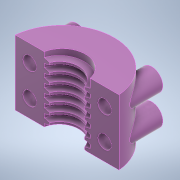
# Autodesk Inventor part: SpindleAdaptor_B_V3
Saved by Autodesk Inventor 2022.2 (Build 262287000, 287)
## iProperties
Created: 2022-11-20
Part Number: SpindleAdaptor_B_V3
Material: ABS Plastic
Document SubType Name: Modeling
Designer: jaege
Density: 1.06 g/cm^3
Appearance: Smooth - Purple
Mass: 4.16051 g
Surface Area: 27.1261 cm^2
Volume: 4.16051 cm^3
Author: jaege
Autodesk Inventor part; units mm, degrees
ref_plane "YZ Plane" through (0, 0, 0) normal (1, 0, 0) x (0, 1, 0)
ref_plane "XZ Plane" through (0, 0, 0) normal (0, 1, 0) x (-1, 0, 0)
ref_plane "XY Plane" through (0, 0, 0) normal (0, 0, 1) x (1, 0, 0)
sketch "Sketch1" plane through (0, 0, 0) normal (0, 1, 0) x (-1, 0, 0)
  circle A0 centre (0, 0) radius 12
  dimension "d0" = 24
  constraints: 1 centre point, 1 coincident
  measures "d0" diameter of A0
extrude "Extrusion1" add sketch "Sketch1" along normal blind 30
sketch "Sketch2" plane through (0, 30, 0) normal (0, 1, 0) x (1, 0, 0)
  circle A0 centre (0, 0) radius 5.25
  dimension "d3" = 10.5
  constraints: 1 centre point, 1 coincident
  measures "d3" diameter of A0
extrude "Extrusion2" cut sketch "Sketch2" against normal blind 15
sketch "Sketch3" plane through (0, 0, 0) normal (0, 0, 1) x (1, 0, 0)
  line L0 (12, 30) -> (-12, 30) projected
  line L1 (12, 0) -> (-12, 0) projected
  line L2 (-5.25, 15) -> (5.25, 15) projected
  line L3 (-5.25, 30) -> (5.25, 30) projected
  line L4 (-5.25, 30) -> (-5.25, 15) projected
  line L5 (5.25, 30) -> (5.25, 15) construction
  line L6 (-5.25, 15) -> (5.25, 15) projected
  line L7 (-4, 15) -> (4, 15) construction
  line L8 (4, 15) -> (4, 30) construction
  line L9 (4, 30) -> (-4, 30) construction
  line L10 (-4, 30) -> (-4, 15) construction
  line L11 (5.25, 30) -> (4, 29.6651)
  line L12 (2.634, 29.299) -> (4, 28.933) construction
  line L13 (4, 29.6651) -> (4, 28.933)
  line L14 (5.25, 28.5981) -> (5.25, 28)
  line L15 (5.25, 28) -> (4, 27.6651)
  line L16 (2.634, 27.299) -> (4, 26.933) construction
  line L17 (4, 29.6651) -> (2.634, 29.299) construction
  line L18 (4, 27.6651) -> (2.634, 27.299) construction
  line L19 (4, 28.933) -> (5.25, 28.5981)
  line L20 (4, 26.933) -> (5.25, 26.5981)
  line L21 (4, 27.6651) -> (4, 26.933)
  line L22 (5.25, 30) -> (5.25, 28.5981)
  line L23 (0, 30) -> (0, 15)
  point P0 (0, 0)
  point P1 (4, 29.299)
  dimension "d6" = 8
  dimension "d7" = 30
  dimension "d8" = 30
  dimension "d9" = 1.25
  dimension "d10" = 105
  dimension "d11" = 105
  dimension "d12" = 0.732
  dimension "d13" = 0.5981
  constraints: 34 end point, 9 point on line, 6 collinear, 3 midpoint, 2 parallel, 2 vertical, 1 horizontal, 1 perpendicular, 1 vertical alignment
  measures "d6" distance between parallel lines of L8 L10
  measures "d7" angle of L12 L11
  measures "d8" angle of L16 L15
  measures "d9" distance between parallel lines of L5 L13
  measures "d10" angle of L5 L11
  measures "d11" angle of L14 L15
  measures "d12" distance of L13.start L12.end
  measures "d13" distance of L14.start L14.end
coil "Coil1" sketch "Sketch3" operation add axis through (0, 30, 0) along (0, -1, 0) pitch 2 turns 7 hand right contours L22 L19 L13 L11
sketch "Sketch4" plane through (0, 0, 0) normal (0, -1, 0) x (1, 0, 0)
  circle A0 centre (0, 0) radius 2
  line L0 (-2, -2) -> (2, -2)
  line L1 (2, -2) -> (2, 1.5)
  line L2 (2, 1.5) -> (-2, 1.5)
  line L3 (-2, 1.5) -> (-2, -2)
  point P0 (1.3229, 1.5)
  point P1 (-1.3229, 1.5)
  dimension "d22" = 4
  dimension "d23" = 3.5
  constraints: 8 end point, 3 tangent, 2 parallel, 1 centre point, 1 coincident, 1 horizontal, 1 perpendicular
  measures "d22" diameter of A0
  measures "d23" distance of L0.end L1.end
extrude "Extrusion3" cut sketch "Sketch4" against normal blind 10 contours A0 L2 picked at (0.2249, -0.4939)
sketch "Sketch5" plane through (0, 0, 0) normal (0, 0, 1) x (1, 0, 0)
  line L0 (12, 30) -> (-12, 30) projected
  line L1 (-5.25, 15) -> (5.25, 15) projected
  line L2 (0, -6) -> (0, 36) projected
  line L3 (-8.625, 26) -> (-12, 26) construction
  line L4 (-8.625, 26) -> (-5.25, 26) construction
  line L5 (-5.25, 30) -> (-5.25, 15) projected
  line L6 (-12, 0) -> (-12, 30) projected
  circle A0 centre (-8.625, 19) radius 1.55
  circle A1 centre (-8.625, 26) radius 1.55
  circle A2 centre (8.625, 26) radius 1.55
  circle A3 centre (8.625, 19) radius 1.55
  point P0 (0, 0)
  point P1 (1.5921, 15)
  dimension "d26" = 4
  dimension "d27" = 4
  dimension "d28" = 3.1
  constraints: 4 centre point, 4 coincident, 4 end point, 4 vertical alignment, 3 equal radius, 2 horizontal, 2 horizontal alignment, 1 collinear, 1 symmetric about line
  measures "d26" distance from line of L0 L3.start
  measures "d27" distance from line of L1 point (-8.625, 19)
  measures "d28" diameter of A0
extrude "Extrusion4" cut sketch "Sketch5" along normal through all both and the other way through all contours A0 | A1 | A2 | A3
ref_plane "Work Plane1" through (0, 0, -12) normal (0, 0, -1) x (-1, 0, 0)
sketch "Sketch6" plane through (0, 0, -12) normal (0, 0, -1) x (-1, 0, 0)
  circle A0 centre (-8.625, 26) radius 1.55
  line L0 (-12, 0) -> (-12, 30) projected
  line L1 (-5.25, 28.5981) -> (-5.25, 30) projected
  line L2 (12, 0) -> (12, 30) projected
  line L3 (12, 30) -> (-12, 30) projected
  line L4 (0, 30) -> (0, 0)
  line L5 (-8.625, 26) -> (-8.625, 29.0718) construction
  line L6 (-8.625, 29.0718) -> (-12, 29.0718) construction
  line L7 (-8.625, 29.0718) -> (-5.25, 29.0718) construction
  line L8 (-5.25, 15) -> (5.25, 15) projected
  circle A1 centre (-8.625, 19) radius 1.55
  circle A2 centre (8.625, 19) radius 1.55
  circle A3 centre (8.625, 26) radius 1.55
  circle A4 centre (8.625, 19) radius 2.55
  circle A5 centre (8.625, 26) radius 2.55
  circle A6 centre (-8.625, 26) radius 2.55
  circle A7 centre (-8.625, 19) radius 2.55
  line L9 (-5.25, 28.5981) -> (-5.25, 0) construction
  line L10 (12, 0) -> (-12, 0) projected
  point P0 (-1.5921, 15)
  dimension "d31" = 3.1
  dimension "d32" = 4
  dimension "d33" = 4
  dimension "d34" = 5.1
  constraints: 10 end point, 8 centre point, 6 equal radius, 4 point on line, 3 coincident, 3 vertical, 2 horizontal alignment, 2 vertical alignment, 1 collinear, 1 midpoint, 1 perpendicular, 1 symmetric about line
  measures "d31" diameter of A0
  measures "d32" distance from line of L5.start L3
  measures "d33" distance from line of L8 A1.centre
  measures "d34" diameter of A7
ref_plane "Work Plane2" through (0, 0, 12) normal (0, 0, -1) x (-1, 0, 0)
extrude "Extrusion5" add sketch "Sketch6" against normal up to surface (24 mm away) contours A4 | A5 | A6 | A7
sketch "Sketch7" plane through (0, 30, 0) normal (0, 1, 0) x (1, 0, 0)
  circle A0 centre (0, 0) radius 12 projected
  line L0 (-16.8, -12) -> (16.8, -12) projected
  line L1 (-12, 0) -> (12, 0)
  line L2 (12, -12) -> (12, 0)
  line L3 (12, -12) -> (-12, -12)
  line L4 (-12, 0) -> (-12, -12)
  constraints: 8 end point, 2 point on circle, 2 point on line, 2 vertical, 1 horizontal, 1 midpoint
extrude "Extrusion6" cut sketch "Sketch7" against normal through all contours L2 L0 A0 | A0 L1 | A0 L0 L4 picked at (2.494, -3.1273)
sketch "Sketch8" plane through (-5.25, 15, 0) normal (0, 0, 1) x (1, 0, 0)
  line L0 (-6.75, -15) -> (-6.75, 15) projected
  line L1 (17.25, -15) -> (17.25, 15) projected
  line L2 (-6.75, 0) -> (17.25, 0)
  line L3 (17.25, 0) -> (17.25, -15)
  line L4 (17.25, -15) -> (-6.75, -15)
  line L5 (-6.75, -15) -> (-6.75, 0)
  point P0 (5.25, -15)
  point P1 (-6.75, -15)
  constraints: 8 end point, 2 parallel, 1 horizontal, 1 midpoint, 1 perpendicular
extrude "Extrusion7" cut sketch "Sketch8" against normal through all
sketch "Sketch9" plane through (5.25, 30, 0) normal (0, 0, 1) x (1, 0, 0)
  line L0 (-17.25, -15) -> (-10.5, -15) projected
  line L1 (-10.5, -14.4019) -> (-10.5, -15) projected
  line L2 (-9.25, -13.3349) -> (-9.25, -14.067) projected
  line L3 (-10.5, -12.4019) -> (-10.5, -13) projected
  line L4 (-9.25, -11.3349) -> (-9.25, -12.067) projected
  line L5 (-10.5, -10.4019) -> (-10.5, -11) projected
  line L6 (-9.25, -9.3349) -> (-9.25, -10.067) projected
  line L7 (-10.5, -8.4019) -> (-10.5, -9) projected
  line L8 (-9.25, -7.3349) -> (-9.25, -8.067) projected
  line L9 (-10.5, -6.4019) -> (-10.5, -7) projected
  line L10 (-9.25, -5.3349) -> (-9.25, -6.067) projected
  line L11 (-10.5, -4.4019) -> (-10.5, -5) projected
  line L12 (-9.25, -3.3349) -> (-9.25, -4.067) projected
  line L13 (-10.5, -2.4019) -> (-10.5, -3) projected
  line L14 (-9.25, -1.3349) -> (-9.25, -2.067) projected
  line L15 (-10.5, 0) -> (-10.5, -1) projected
  line L16 (-17.25, 0) -> (-10.5, 0) projected
  line L17 (-17.25, -15) -> (-17.25, 0) projected
  circle A0 centre (-13.875, -4) radius 1.55 projected
  circle A1 centre (-13.875, -11) radius 1.55 projected
  circle A2 centre (3.375, -4) radius 1.55 projected
  circle A3 centre (3.375, -11) radius 1.55 projected
  line L18 (-1.25, -15) -> (6.75, -15) projected
  line L19 (6.75, -15) -> (6.75, 0) projected
  line L20 (0, 0) -> (6.75, 0) projected
  line L21 (0, -2) -> (0, 0) projected
  line L22 (-1.25, -3.067) -> (-1.25, -2.3349) projected
  line L23 (0, -4) -> (0, -3.4019) projected
  line L24 (-1.25, -5.067) -> (-1.25, -4.3349) projected
  line L25 (0, -6) -> (0, -5.4019) projected
  line L26 (-1.25, -7.067) -> (-1.25, -6.3349) projected
  line L27 (0, -8) -> (0, -7.4019) projected
  line L28 (-1.25, -9.067) -> (-1.25, -8.3349) projected
  line L29 (0, -10) -> (0, -9.4019) projected
  line L30 (-1.25, -11.067) -> (-1.25, -10.3349) projected
  line L31 (0, -12) -> (0, -11.4019) projected
  line L32 (-1.25, -13.067) -> (-1.25, -12.3349) projected
  line L33 (0, -14) -> (0, -13.4019) projected
  line L34 (0, -14) -> (-1.25, -14.3349) projected
  line L35 (-1.25, -14.3349) -> (-1.25, -15) projected
  line L36 (-17.25, 0) -> (6.75, 0)
  line L37 (6.75, 0) -> (6.75, -15)
  line L38 (6.75, -15) -> (-17.25, -15)
  line L39 (-17.25, -15) -> (-17.25, 0)
  point P0 (-5.25, -30)
  constraints: 8 end point, 2 parallel, 1 horizontal, 1 perpendicular, 30 other
extrude "Extrusion8" cut sketch "Sketch9" against normal blind 1 contours L17 L16 L36 L20 L19 L18 L38 L0 | A0 | A1 | A2 | A3
thicken "Thicken1" operation add thickness 0.15 both sides no extend neighbours yes toward (0.638285, 0, -0.7698001) faces at (2.5532, 17.4567, -3.0792) (-2.1727, 18.5368, -4.3175) (3.7195, 18.4487, -3.7051) (-2.1727, 19.3581, -4.3175) (-2.1727, 17.3581, -4.3175) (3.7195, 16.4487, -3.7051) (2.5532, 19.4567, -3.0792) (-2.1727, 20.5368, -4.3175) (-2.1727, 16.5368, -4.3175) (2.3077, 15.7253, -3.2672) (3.3982, 20.6746, -4.0019) (-2.1727, 21.3581, -4.3175) (-4.6344, 15.6181, -1.3725) (-5.0632, 15.3339, -1.3881) (2.5532, 21.4567, -3.0792) (-2.1727, 22.5368, -4.3175) (4.3314, 28.7887, -2.9668) (3.7195, 22.4487, -3.7051) (-2.1727, 23.3581, -4.3175) (-2.1727, 28.5368, -4.3175) (2.5532, 23.4567, -3.0792) (-2.1727, 24.5368, -4.3175) (3.3982, 24.6746, -4.0019) (-2.1727, 25.3581, -4.3175) (2.5532, 25.7007, -3.0792) (-2.1727, 26.5368, -4.3175) (3.7195, 26.4487, -3.7051) (2.5532, 27.7007, -3.0792) (-2.1727, 27.3581, -4.3175) (11.3488, 21.457, -1) (-11.3488, 23.543, -1)
body "Solid1"
